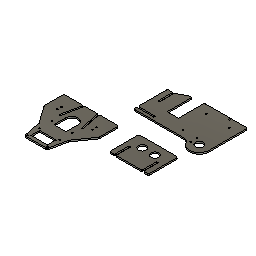
2425-SACBOT-LINE v17 (Autodesk Fusion 360 design; units mm, degrees)
Autodesk Fusion 360 part; units mm, degrees
sketch "Plate Alpha" plane through (0, 0, 0) normal (0, 0, 1) x (1, 0, 0)
  line L0 (0, 0) -> (-55.9249, 0)
  line L1 (-55.9249, 0) -> (-55.9249, -40)
  line L2 (-55.9249, -40) -> (-20.5, -90)
  line L3 (-20.5, -90) -> (0, -90) construction
  line L4 (0, 0) -> (0, -90) construction
  circle A0 centre (-35.9249, -25) radius 1.5
  circle A1 centre (-35.9249, -33) radius 1.5
  line L5 (-35.9249, -25) -> (-35.9249, -33)
  line L6 (0, -59.3106) -> (-20.5, -59.3106) construction
  circle A2 centre (-20.5, -59.3106) radius 1.5
  line L7 (-20.5, -59.3106) -> (-20.5, -84.8106) construction
  circle A3 centre (-20.5, -84.8106) radius 1.5
  line L8 (-23.3833, -41.6168) -> (0, 70.9808) construction
  line L9 (-21.9147, -41.9218) -> (1.4687, 70.6758)
  line L10 (-24.852, -41.3118) -> (-1.4687, 71.2858)
  line L11 (-24.852, -41.3118) -> (-21.9147, -41.9218)
  line L12 (-1.4687, 71.2858) -> (1.4687, 70.6758)
  circle A4 centre (-40.9249, -15) radius 5
  circle A5 centre (20.5, -59.3106) radius 1.5
  line L13 (21.9147, -41.9218) -> (-1.4687, 70.6758)
  line L14 (24.852, -41.3118) -> (1.4687, 71.2858)
  line L15 (24.852, -41.3118) -> (21.9147, -41.9218)
  circle A6 centre (35.9249, -33) radius 1.5
  circle A7 centre (40.9249, -15) radius 5
  line L16 (55.9249, -40) -> (20.5, -90)
  line L17 (20.5, -90) -> (0, -90) construction
  circle A8 centre (20.5, -84.8106) radius 1.5
  line L18 (1.4687, 71.2858) -> (-1.4687, 70.6758)
  circle A9 centre (35.9249, -25) radius 1.5
  circle A10 centre (0, -40) radius 12.5
  line L19 (20.5, -84.8106) -> (0, -84.8106) construction
  line L20 (-20.5, -84.8106) -> (0, -84.8106) construction
  line L21 (-31.6847, -74.2135) -> (-24.852, -41.3118) construction
  line L22 (-21.9147, -41.9218) -> (-29.3153, -77.5578) construction
  line L23 (-23.3833, -41.6168) -> (-30.5, -75.8856) construction
  circle A11 centre (-35.9249, -33) radius 3 construction
  line L24 (-12.5, -63.8106) -> (-12.5, -40)
  line L25 (-12.5, -63.8106) -> (0, -63.8106)
  line L26 (12.5, -63.8106) -> (12.5, -40)
  line L27 (12.5, -63.8106) -> (0, -63.8106)
  line L28 (55.9249, 0) -> (55.9249, -40)
  line L29 (0, 0) -> (55.9249, 0)
  line L30 (23.3833, -41.6168) -> (30.5, -75.8856) construction
  circle A12 centre (-20.5, -84.8106) radius 3 construction
  line L31 (-27.9924, -63.8106) -> (27.9924, -63.8106) construction
  circle A13 centre (-20.5, -59.3106) radius 3 construction
  line L32 (-27.9397, -62.3106) -> (28.362, -62.3106) construction
  line L33 (-37.9924, -65.3106) -> (28.1509, -65.3106) construction
  circle A14 centre (-18.1162, -1.5) radius 1.5
  circle A15 centre (-11.9882, -1.5) radius 1.5
  circle A16 centre (11.9882, -1.5) radius 1.5
  circle A17 centre (18.1162, -1.5) radius 1.5
  line L34 (-20.5, -84.8106) -> (-20.5, -109.8106) construction
  line L35 (-20.5, -109.8106) -> (0, -109.8106) construction
  circle A18 centre (-20.5, -109.8106) radius 1.5
  line L36 (-23.5, -84.8106) -> (-23.5, -112.8106)
  line L37 (-23.5, -112.8106) -> (0, -112.8106)
  line L38 (23.5, -84.8106) -> (23.5, -112.8106)
  line L39 (23.5, -112.8106) -> (0, -112.8106)
  circle A19 centre (20.5, -109.8106) radius 1.5
  circle A20 centre (-20.5, -109.8106) radius 3
  circle A21 centre (20.5, -109.8106) radius 3
  line L40 (-16.75, -88.5606) -> (-16.75, -106.0606)
  line L41 (-16.75, -106.0606) -> (0, -106.0606)
  line L42 (-16.75, -88.5606) -> (0, -88.5606)
  line L43 (16.75, -88.5606) -> (0, -88.5606)
  line L44 (16.75, -88.5606) -> (16.75, -106.0606)
  line L45 (16.75, -106.0606) -> (0, -106.0606)
  line L46 (23.4392, -110.4117) -> (30.5, -75.8856)
  line L47 (-30.5, -75.8856) -> (-23.4392, -110.4117)
  point P0 (-55.9249, 0)
  point P1 (20.5, -84.8106)
  point P2 (-28.3039, -65.3106)
  point P3 (-14.7407, 0)
  point P4 (20.5, -109.8106)
  dimension "d123" = 3
  dimension "d124" = 3
  dimension "d125" = 20
  dimension "d126" = 8
  dimension "d127" = 20.5
  dimension "d128" = 3
  dimension "d129" = 25.5
  dimension "d130" = 3
  dimension "d131" = 1.5
  dimension "d132" = -1.5
  dimension "d133" = 10
  dimension "d135" = 25
  dimension "d136" = 40
  dimension "d137" = 50
  dimension "d143" = 35
  dimension "d144" = 115
  dimension "d146" = 6
  dimension "d147" = 10
  dimension "d148" = 15
  dimension "d149" = 15
  dimension "d150" = 50
  dimension "d165" = 6
  dimension "d167" = 6
  dimension "d168" = -1.5
  dimension "d169" = 1.5
  dimension "d170" = 10
  dimension "d171" = 25
  dimension "d214" = 3
  dimension "d215" = 3
  dimension "d243" = 25
  dimension "d244" = 3
  dimension "d245" = 3
  dimension "d246" = 6
  dimension "d247" = 6
  dimension "d272" = 6.75
  dimension "d274" = 3.75
  dimension "d275" = 6.75
  constraint horizontal L0
  constraint perpendicular L0 L1
  constraint parallel L0 L3
  constraint vertical L4
  constraint coincident L0.start L4.start
  constraint coincident L3.end L4.end
  constraint coincident A0.centre L5.start
  constraint coincident A1.centre L5.end
  constraint vertical L5
  constraint coincident L4 L6.start
  constraint perpendicular L4 L6
  constraint coincident L6.end A2.centre
  constraint perpendicular L6 L7
  constraint coincident L7.end A3.centre
  constraint coincident L4 L8.end
  constraint perpendicular L9 L11
  constraint perpendicular L9 L12
  constraint coincident L8.end L12
  constraint symmetric L1.end L4 L16.start
  constraint symmetric L2.end L4 L16.end
  constraint symmetric L3.end L4 L17.end
  constraint symmetric L4 A1 A6
  constraint symmetric L4 A2 A5
  constraint symmetric L4 L7.end P1
  constraint symmetric L4 A3 A8
  constraint symmetric L4 L9.start L13.start
  constraint symmetric L4 L9.end L13.end
  constraint symmetric L4 L10.start L14.start
  constraint symmetric L4 L10.end L14.end
  constraint symmetric L4 A4 A7
  constraint coincident L2.end L7
  constraint coincident L8.start L11
  constraint symmetric L4 A0 A9
  constraint coincident L4 A10.centre
  constraint coincident L2 L21.start
  constraint coincident L2 L22.end
  constraint collinear L10 L21
  constraint collinear L9 L22
  constraint coincident L2 L23.end
  constraint parallel L22 L23
  constraint coincident P0 L1
  constraint coincident P0 L0
  constraint concentric A1 A11
  constraint coincident A10 L24.end
  constraint tangent A10 L24
  constraint coincident L4 L25.end
  constraint perpendicular L4 L25
  constraint coincident L24.start L25
  constraint vertical L24
  constraint symmetric L4 L24.start L26.start
  constraint symmetric L4 L24.end L26.end
  constraint symmetric L4 L25.end L27.end
  constraint coincident L1 P0
  constraint coincident P0 L0.end
  constraint symmetric L0.start L4 L29.start
  constraint symmetric L4 P0 L28.start
  constraint symmetric L4 L8.start L30.start
  constraint symmetric L4 L23.end L30.end
  constraint concentric A3 A12
  constraint tangent L2 A12
  constraint coincident L23 L31.start
  constraint coincident L30 L31.end
  constraint perpendicular L24 L31
  constraint concentric A2 A13
  constraint horizontal L33
  constraint coincident L2 L33.start
  constraint tangent A13 L32
  constraint coincident L33 P2
  constraint coincident L23 P2
  constraint coincident L8 P3
  constraint coincident L0 P3
  constraint tangent L0 A14
  constraint tangent L10 A14
  constraint tangent L9 A15
  constraint tangent L0 A15
  constraint symmetric L4 A14 A17
  constraint symmetric L4 A15 A16
  constraint perpendicular L20 L34
  constraint perpendicular L34 L35
  constraint coincident L4 L35.end
  constraint coincident L34.end L35.start
  constraint symmetric L4 L34.end P4
  constraint symmetric L4 A18 A19
  constraint symmetric L4 L36.start L38.start
  constraint symmetric L4 L36.end L38.end
  constraint symmetric L4 L37.end L39.end
  constraint concentric A18 A20
  constraint concentric A19 A21
  constraint coincident L25.end L31
  constraint coincident L24.start L25.start
  constraint perpendicular L3 L40
  constraint perpendicular L40 L41
  constraint coincident L4 L42.end
  constraint perpendicular L4 L42
  constraint coincident L4 L41.end
  constraint symmetric L4 L40.start L43.start
  constraint symmetric L4 L40.end L44.end
  constraint symmetric L4 L41.end L45.end
  constraint symmetric L4 L42.end L43.end
  constraint coincident A21 L46.start
  constraint tangent A21 L46
  constraint coincident A20 L47.end
  constraint tangent A20 L47
  measures "d123" diameter of A0
  measures "d124" diameter of A1
  measures "d125" distance of L1 L5
  measures "d126" distance of A0.centre A1.centre
  measures "d127" distance of L6.start L6.end
  measures "d128" diameter of A2
  measures "d129" distance of L6.end L7.end
  measures "d130" diameter of A3
  measures "d133" diameter of A4
  measures "d135" diameter of A10
  measures "d136" distance of P0 L1.end
  measures "d137" vertical distance of L1.end L2.end
  measures "d143" distance of L8.start L23.end
  measures "d144" distance of L8.start L8.end
  measures "d146" diameter of A11
  measures "d147" horizontal distance of L2.end L23.end
  measures "d148" distance of L1 A4.centre
  measures "d149" distance of L0 A4.centre
  measures "d150" distance of L3.end A10.centre
  measures "d165" diameter of A12
  measures "d167" diameter of A13
  measures "d170" horizontal distance of L31.start L33.start
  measures "d171" distance of L0 A0.centre
  measures "d214" diameter of A15
  measures "d215" diameter of A14
  measures "d243" distance of L7.end L34.end
  measures "d244" diameter of A18
  measures "d246" diameter of A20
  measures "d247" diameter of A21
  measures "d272" distance of L36 L40
  measures "d274" distance of L20 L42
  measures "d275" distance of L37 L41
sketch "Plate Gamma" plane through (0, 0, 0) normal (0, 0, 1) x (1, 0, 0)
  line L0 (-279.3639, -68.2725) -> (-160.8639, -68.2725)
  line L1 (-160.8639, -68.2725) -> (-160.8639, -118.2725)
  line L2 (-160.8639, -118.2725) -> (-279.3639, -118.2725)
  line L3 (-279.3639, -118.2725) -> (-279.3639, -68.2725)
  line L4 (-220.1139, -68.2725) -> (-220.1139, -118.2725) construction
  circle A0 centre (-233.1139, -93.2725) radius 8
  line L5 (-233.1139, -85.2725) -> (-220.1139, -85.2725)
  line L6 (-233.1139, -101.2725) -> (-220.1139, -101.2725)
  line L7 (-264.3639, -118.2725) -> (-264.3639, -93.2725)
  line L8 (-262.1639, -120.6703) -> (-262.1639, -95.6703)
  line L9 (-266.5639, -120.6703) -> (-266.5639, -95.6703)
  line L10 (-266.5639, -95.6703) -> (-262.1639, -95.6703)
  line L11 (-279.3639, -93.2725) -> (-160.8639, -93.2725) construction
  circle A1 centre (-207.1139, -93.2725) radius 8
  line L12 (-207.1139, -85.2725) -> (-220.1139, -85.2725)
  line L13 (-207.1139, -101.2725) -> (-220.1139, -101.2725)
  line L14 (-178.0639, -120.6703) -> (-178.0639, -95.6703)
  line L15 (-173.6639, -120.6703) -> (-173.6639, -95.6703)
  line L16 (-173.6639, -95.6703) -> (-178.0639, -95.6703)
  arc A2 (-262.1639, -115.2725) -> (-259.1639, -118.2725) centre (-259.1639, -115.2725) ccw
  arc A3 (-269.5639, -118.2725) -> (-266.5639, -115.2725) centre (-269.5639, -115.2725) ccw
  arc A4 (-181.0639, -118.2725) -> (-178.0639, -115.2725) centre (-181.0639, -115.2725) ccw
  arc A5 (-173.6639, -115.2725) -> (-170.6639, -118.2725) centre (-170.6639, -115.2725) ccw
  line L17 (-39.7924, -33.8106) -> (-39.7924, -93.8106)
  line L18 (-39.7924, -93.8106) -> (39.7924, -93.8106)
  line L19 (39.7924, -93.8106) -> (39.7924, -33.8106)
  line L20 (39.7924, -33.8106) -> (-39.7924, -33.8106)
  circle A6 centre (-12.75, -53.8106) radius 7.925
  line L21 (0, -33.8106) -> (0, -93.8106) construction
  line L22 (-12.75, -45.8856) -> (0, -45.8856)
  line L23 (-12.75, -61.7356) -> (0, -61.7356)
  line L24 (-27.9924, -63.8106) -> (27.9924, -63.8106)
  circle A7 centre (12.75, -53.8106) radius 7.925
  line L25 (12.75, -45.8856) -> (0, -45.8856)
  line L26 (12.75, -61.7356) -> (0, -61.7356)
  line L27 (-4.5784, -44.6359) -> (0, -44.6359)
  line L28 (0, -44.6359) -> (0, -33.8106)
  line L29 (-27.9924, -63.8106) -> (-27.9924, -93.8106) construction
  line L30 (-29.7924, -63.8106) -> (-29.7924, -93.8106)
  line L31 (-26.1924, -63.8106) -> (-26.1924, -93.8106)
  line L32 (-29.7924, -63.8106) -> (-26.1924, -63.8106)
  line L33 (27.9924, -63.8106) -> (27.9924, -93.8106) construction
  line L34 (-26.1924, -63.8106) -> (-12.75, -53.8106)
  circle A8 centre (-24.6924, -92.3106) radius 1.5
  circle A9 centre (-31.2924, -92.3106) radius 1.5
  circle A10 centre (24.6924, -92.3106) radius 1.5
  circle A11 centre (31.2924, -92.3106) radius 1.5
  line L35 (29.7924, -63.8106) -> (29.7924, -93.8106)
  line L36 (26.1924, -63.8106) -> (26.1924, -93.8106)
  line L37 (29.7924, -63.8106) -> (26.1924, -63.8106)
  point P0 (-19.1085, -58.5409)
  dimension "d29" = 2.2
  dimension "d30" = -2.2
  dimension "d31" = 16
  dimension "d32" = 25
  dimension "d33" = 13
  dimension "d34" = 44.25
  dimension "d39" = 15
  dimension "d68" = 3
  dimension "d69" = 6
  dimension "d178" = 15.85
  dimension "d182" = 1.8
  dimension "d183" = -1.8
  dimension "d186" = 10
  dimension "d189" = 60
  dimension "d230" = 3
  dimension "d231" = 3
  dimension "d248" = 20
  dimension "d249" = 30
  dimension "d250" = 25.5
  constraint horizontal L0
  constraint vertical L1
  constraint horizontal L2
  constraint vertical L3
  constraint midpoint L0 L4.start
  constraint midpoint L2 L4.end
  constraint coincident A0 L5.start
  constraint coincident L4 L5.end
  constraint horizontal L5
  constraint tangent A0 L5
  constraint coincident A0 L6.start
  constraint coincident L4 L6.end
  constraint horizontal L6
  constraint tangent A0 L6
  constraint coincident L2 L7.start
  constraint perpendicular L2 L7
  constraint perpendicular L8 L10
  constraint midpoint L3 L11.start
  constraint midpoint L1 L11.end
  constraint coincident A0.centre L11
  constraint coincident L7.end L11
  constraint symmetric L4 A0 A1
  constraint symmetric L4 L5.start L12.start
  constraint symmetric L4 L5.end L12.end
  constraint symmetric L4 L6.start L13.start
  constraint symmetric L4 L6.end L13.end
  constraint symmetric L4 L8.start L14.start
  constraint symmetric L4 L8.end L14.end
  constraint symmetric L4 L9.start L15.start
  constraint symmetric L4 L9.end L15.end
  constraint tangent L2 A2
  constraint tangent L8 A2
  constraint coincident L2 A2.end
  constraint coincident L8 A2.start
  constraint tangent L2 A3
  constraint tangent L9 A3
  constraint coincident L9 A3.end
  constraint coincident L2 A3.start
  constraint symmetric L4 A2.end A4.start
  constraint symmetric L4 A2.start A4.end
  constraint symmetric L4 A2 A4
  constraint symmetric L4 A3.end A5.start
  constraint symmetric L4 A3.start A5.end
  constraint symmetric L4 A3 A5
  constraint vertical L17
  constraint perpendicular L17 L18
  constraint perpendicular L18 L19
  constraint midpoint L20 L21.start
  constraint midpoint L18 L21.end
  constraint perpendicular L18 L21
  constraint coincident A6 L22.start
  constraint coincident L21 L22.end
  constraint tangent A6 L22
  constraint perpendicular L21 L22
  constraint coincident A6 L23.start
  constraint coincident L21 L23.end
  constraint tangent A6 L23
  constraint perpendicular L21 L23
  constraint symmetric A6 L21 A7
  constraint symmetric L21 L22.start L25.start
  constraint symmetric L21 L22.end L25.end
  constraint symmetric L21 L23.start L26.start
  constraint symmetric L21 L23.end L26.end
  constraint horizontal L20
  constraint horizontal L27
  constraint coincident L20 L21.start
  constraint perpendicular L20 L28
  constraint midpoint L21 L24
  constraint coincident L24.start L29.start
  constraint coincident L18 L29.end
  constraint perpendicular L18 L29
  constraint perpendicular L31 L32
  constraint coincident L24.end L33.start
  constraint coincident L18 L33.end
  constraint perpendicular L18 L33
  constraint coincident A6.centre L34.end
  constraint coincident A6 P0
  constraint coincident L34 P0
  constraint coincident L18 L31.end
  constraint coincident L18 L30.end
  constraint tangent L30 A9
  constraint tangent L18 A9
  constraint tangent L31 A8
  constraint tangent L18 A8
  constraint symmetric L21 A8 A10
  constraint symmetric L21 A9 A11
  constraint symmetric L21 L30.start L35.start
  constraint symmetric L21 L30.end L35.end
  constraint symmetric L21 L31.start L36.start
  constraint symmetric L21 L31.end L36.end
  measures "d31" diameter of A0
  measures "d32" distance of L2 A0.centre
  measures "d33" distance of L4 A0.centre
  measures "d34" distance of L4 L7.start
  measures "d39" distance of L7.end L11.start
  measures "d68" radius of A2
  measures "d69" diameter of A3
  measures "d178" diameter of A6
  measures "d186" distance of L17 L30
  measures "d189" distance of L17.start L17.end
  measures "d230" diameter of A8
  measures "d231" diameter of A9
  measures "d248" distance of L20 A6.centre
  measures "d249" distance of L30.start L30.end
  measures "d250" distance of A7.centre A6.centre
sketch "Plate Beta" plane through (0, 0, 0) normal (0, 0, 1) x (1, 0, 0)
  line L0 (48.3507, -123.1753) -> (48.3507, -73.1753)
  line L1 (48.3507, -73.1753) -> (193.8507, -73.1753)
  line L2 (193.8507, -73.1753) -> (193.8507, -146.3349)
  line L3 (68.8507, -146.1753) -> (68.8507, -123.1753)
  line L4 (68.8507, -123.1753) -> (48.3507, -123.1753)
  line L5 (68.8507, -73.1753) -> (68.8507, -98.1753)
  line L6 (66.6507, -73.7918) -> (66.6507, -98.7918)
  line L7 (71.0507, -73.7918) -> (71.0507, -98.7918)
  line L8 (66.6507, -98.7918) -> (71.0507, -98.7918)
  line L9 (68.8507, -123.1753) -> (93.8507, -123.1753)
  line L10 (93.8507, -123.1753) -> (93.8507, -126.1753)
  line L11 (93.8507, -126.1753) -> (68.8507, -126.1753)
  arc A0 (66.6507, -76.1753) -> (63.6507, -73.1753) centre (63.6507, -76.1753) ccw
  arc A1 (74.0507, -73.1753) -> (71.0507, -76.1753) centre (74.0507, -76.1753) ccw
  arc A2 (71.8507, -126.1753) -> (68.8507, -129.1753) centre (71.8507, -129.1753) ccw
  arc A3 (142.4447, -171.4545) -> (193.8507, -146.3349) centre (162.0103, -146.3349) ccw
  line L12 (83.4734, -73.1753) -> (83.4734, -159.2628) construction
  line L13 (83.4734, -116.2191) -> (95.5231, -116.2191) construction
  line L14 (95.5231, -116.2191) -> (180.6062, -116.2191) construction
  circle A4 centre (83.4734, -116.2191) radius 4.5
  line L15 (111.0507, -57.3516) -> (111.0507, -183.7559) construction
  line L16 (93.8507, -123.1753) -> (193.8507, -123.1753) construction
  line L17 (125.0507, -57.3516) -> (125.0507, -183.7559) construction
  line L18 (177.1507, -57.3516) -> (177.1507, -183.7559) construction
  line L19 (95.9516, -120.6753) -> (195.9516, -120.6753) construction
  line L20 (95.9516, -115.5753) -> (195.9516, -115.5753) construction
  line L21 (95.9516, -87.6753) -> (195.9516, -87.6753) construction
  circle A5 centre (125.0507, -120.6753) radius 1.5
  circle A6 centre (177.1507, -115.5753) radius 1.5
  circle A7 centre (177.1507, -87.6753) radius 1.5
  circle A8 centre (159.8734, -146.2859) radius 8
  line L22 (119.02, -178.1753) -> (211.8685, -178.1753)
  arc A9 (142.4447, -171.4545) -> (68.8507, -146.1753) centre (68.8507, -265.9397) ccw
  line L23 (68.8507, -146.1753) -> (95.1653, -146.1753) construction
  line L24 (-23.3833, -41.6168) -> (0, 70.9808)
  line L25 (-23.3833, -41.6168) -> (-30.5, -75.8856)
  circle A10 centre (171.8682, 109.4824) radius 1.5
  circle A11 centre (123.6682, 110.7824) radius 1.5
  circle A12 centre (128.7682, 58.6824) radius 1.5
  circle A13 centre (156.6682, 58.6824) radius 1.5
  line L26 (156.6682, 58.6824) -> (128.7682, 58.6824) construction
  line L27 (174.4682, 124.7824) -> (121.1682, 124.7824) construction
  line L28 (121.1682, 124.7824) -> (121.1682, 56.1824) construction
  line L29 (121.1682, 56.1824) -> (174.4682, 56.1824) construction
  line L30 (174.4682, 56.1824) -> (174.4682, 124.7824) construction
  line L31 (-39.7924, -33.8106) -> (-39.7924, -93.8106)
  line L32 (-27.9924, -63.8106) -> (-27.9924, -93.8106)
  line L33 (41.1416, 114.4163) -> (41.1416, 54.4163)
  line L34 (41.1416, 54.4163) -> (76.1416, 54.4163)
  line L35 (76.1416, 54.4163) -> (76.1416, 51.4163)
  line L36 (76.1416, 51.4163) -> (41.1416, 51.4163)
  line L37 (41.1416, 51.4163) -> (41.1416, 29.4163)
  line L38 (41.1416, 114.4163) -> (51.8242, 114.4163)
  line L39 (51.8242, 114.4163) -> (51.8242, 84.4163)
  line L40 (51.8242, 84.4163) -> (55.1242, 84.4163)
  line L41 (55.1242, 84.4163) -> (55.1242, 114.4163)
  line L42 (191.1416, 127.4163) -> (191.1416, 29.4163)
  line L43 (55.1242, 114.4163) -> (80.2572, 127.4163)
  line L44 (80.2572, 127.4163) -> (191.1416, 127.4163)
  line L45 (191.1416, 29.4163) -> (41.1416, 29.4163)
  line L46 (118.6464, 29.4163) -> (118.6464, 127.4163) construction
  circle A14 centre (171.1416, 49.4163) radius 20
  line L47 (41.1416, 45.4163) -> (143.7995, 45.4163)
  arc A15 (153.7053, 39.6197) -> (143.7995, 45.4163) centre (143.7995, 34.0541) ccw
  circle A16 centre (56.6242, 113.5034) radius 1.5
  circle A17 centre (50.3242, 112.9163) radius 1.5
  circle A18 centre (171.1416, 49.4163) radius 8
  line L48 (80.2572, 127.4163) -> (80.2572, 74.4163)
  line L49 (80.2572, 74.4163) -> (103.2572, 74.4163)
  line L50 (103.2572, 74.4163) -> (103.2572, 127.4163)
  line L51 (157.2609, 45.7074) -> (157.2609, 123.8574) construction
  circle A19 centre (157.2609, 45.7074) radius 1.5
  circle A20 centre (157.2609, 45.7074) radius 5.9 construction
  circle A21 centre (157.2609, 123.8574) radius 1.5
  circle A22 centre (157.2609, 123.8574) radius 5.9 construction
  line L52 (130.7609, 44.7824) -> (183.7609, 44.7824) construction
  line L53 (183.7609, 44.7824) -> (183.7609, 124.7824) construction
  line L54 (183.7609, 124.7824) -> (130.7609, 124.7824) construction
  line L55 (130.7609, 124.7824) -> (130.7609, 44.7824) construction
  line L56 (130.7609, 44.7824) -> (183.7609, 124.7824) construction
  point P0 (53.4742, 84.4163)
  point P1 (-14.7407, 0)
  point P2 (41.1416, 45.4163)
  dimension "d17" = 2.2
  dimension "d18" = -2.2
  dimension "d19" = 25
  dimension "d20" = 50
  dimension "d21" = 3
  dimension "d22" = 25
  dimension "d25" = 20.5
  dimension "d26" = 20.5
  dimension "d27" = 100
  dimension "d28" = 20
  dimension "d64" = 3
  dimension "d65" = 6
  dimension "d66" = 3
  dimension "d80" = 9
  dimension "d81" = 40
  dimension "d82" = -14
  dimension "d83" = -66.1
  dimension "d84" = -2.5
  dimension "d85" = -7.6
  dimension "d86" = -35.5
  dimension "d87" = 3
  dimension "d88" = 3
  dimension "d89" = 3
  dimension "d90" = 16
  dimension "d115" = 55
  dimension "d151" = 3
  dimension "d152" = 3
  dimension "d153" = 3
  dimension "d154" = 3
  dimension "d157" = 27.9
  dimension "d160" = 68.6
  dimension "d161" = 53.3
  dimension "d162" = 2.5
  dimension "d163" = 14
  dimension "d190" = 115
  dimension "d191" = 35
  dimension "d192" = 60
  dimension "d193" = 30
  dimension "d195" = 12.3326
  dimension "d196" = 12.3326
  dimension "d197" = 3.3
  dimension "d198" = 115
  dimension "d199" = 60
  dimension "d200" = 30
  dimension "d202" = 3
  dimension "d203" = 25
  dimension "d204" = 72.4953
  dimension "d205" = 72.4953
  dimension "d206" = 6
  dimension "d207" = 3
  dimension "d208" = 3
  dimension "d211" = 35
  dimension "d212" = 40
  dimension "d213" = 16
  dimension "d251" = 23
  dimension "d252" = 53
  dimension "d253" = 20
  dimension "d256" = 5.1
  dimension "d257" = 15.2
  dimension "d258" = 1.3
  dimension "d259" = 50.8
  dimension "d260" = 78.15
  dimension "d261" = 80
  dimension "d262" = 3
  dimension "d263" = 11.8
  dimension "d264" = 3
  dimension "d265" = 11.8
  dimension "d266" = 53
  dimension "d267" = 180
  constraint vertical L0
  constraint perpendicular L0 L1
  constraint perpendicular L1 L2
  constraint parallel L2 L3
  constraint horizontal L4
  constraint coincident L1 L5.start
  constraint perpendicular L1 L5
  constraint perpendicular L7 L8
  constraint perpendicular L3 L9
  constraint perpendicular L9 L10
  constraint coincident L3 L11.end
  constraint horizontal L11
  constraint tangent L1 A0
  constraint tangent L6 A0
  constraint coincident L1 A0.end
  constraint coincident L6 A0.start
  constraint tangent L7 A1
  constraint tangent L1 A1
  constraint coincident L7 A1.end
  constraint coincident L1 A1.start
  constraint tangent L3 A2
  constraint tangent L11 A2
  constraint coincident L3 A2.end
  constraint coincident L11 A2.start
  constraint tangent L2 A3
  constraint coincident L1 L12.start
  constraint perpendicular L1 L12
  constraint midpoint L12 L13.start
  constraint perpendicular L12 L13
  constraint perpendicular L12 L14
  constraint coincident L13.start A4.centre
  constraint vertical L15
  constraint coincident L2 L16.end
  constraint horizontal L16
  constraint coincident L17 A5.centre
  constraint coincident L19 A5.centre
  constraint coincident L20 A6.centre
  constraint coincident L18 A6.centre
  constraint coincident L21 A7.centre
  constraint coincident L18 A7.centre
  constraint horizontal L22
  constraint tangent A3 L22
  constraint tangent A3 A9
  constraint perpendicular L3 L23
  constraint tangent A9 L23
  constraint coincident A13.centre L26.start
  constraint coincident A12.centre L26.end
  constraint perpendicular L27 L28
  constraint perpendicular L28 L29
  constraint coincident L27.start L30.end
  constraint vertical L18
  constraint vertical L33
  constraint perpendicular L33 L34
  constraint perpendicular L34 L35
  constraint perpendicular L35 L36
  constraint perpendicular L36 L37
  constraint perpendicular L33 L38
  constraint perpendicular L38 L39
  constraint perpendicular L33 L40
  constraint perpendicular L38 L41
  constraint perpendicular L38 L42
  constraint midpoint L40 P0
  constraint collinear L33 L37
  constraint coincident L42.start L44.end
  constraint horizontal L44
  constraint coincident L38 L41.end
  constraint perpendicular L42 L45
  constraint coincident L37.end L45.end
  constraint coincident L45 L46.start
  constraint coincident L44 L46.end
  constraint perpendicular L44 L46
  constraint coincident L37 P2
  constraint tangent L42 A14
  constraint tangent L45 A14
  constraint coincident P2 L47.start
  constraint perpendicular L37 L47
  constraint coincident A14 A15.start
  constraint tangent L47 A15
  constraint tangent A14 A15
  constraint tangent L41 A16
  constraint tangent L43 A16
  constraint tangent L39 A17
  constraint tangent L38 A17
  constraint coincident A14.centre A18.centre
  constraint coincident L44 L43.end
  constraint perpendicular L44 L48
  constraint perpendicular L41 L49
  constraint coincident L44 L50.end
  constraint perpendicular L44 L50
  constraint coincident L43.end L48
  constraint perpendicular L27 L30
  constraint vertical L30
  constraint parallel L26 L29
  constraint coincident L51.start A19.centre
  constraint concentric A19 A20
  constraint coincident L51.end A21.centre
  constraint concentric A21 A22
  constraint perpendicular L53 L54
  constraint midpoint L51 L56
  constraint perpendicular L52 L55
  constraint perpendicular L54 L55
  constraint parallel L51 L55
  measures "d19" distance of L5.start L5.end
  measures "d20" distance of L0.start L0.end
  measures "d21" distance of L9.end L10.end
  measures "d22" distance of L10.end L11.end
  measures "d25" distance of L0.start L3.end
  measures "d26" distance of L0 L5
  measures "d27" distance of L2 L9.end
  measures "d28" distance of L3.start L11.end
  measures "d64" radius of A0
  measures "d65" diameter of A1
  measures "d66" radius of A2
  measures "d80" diameter of A4
  measures "d81" distance of L7 L15
  measures "d87" diameter of A5
  measures "d88" diameter of A6
  measures "d89" diameter of A7
  measures "d90" diameter of A8
  measures "d115" distance of L9.end L22
  measures "d151" diameter of A10
  measures "d152" diameter of A11
  measures "d153" diameter of A12
  measures "d154" diameter of A13
  measures "d157" distance of A13.centre A12.centre
  measures "d160" distance of L27.end L28.end
  measures "d161" distance of L27.start L27.end
  measures "d162" distance of A11.centre L28
  measures "d163" distance of A11.centre L27
  measures "d190" distance of L24.start L24.end
  measures "d191" distance of L24.start L25.end
  measures "d192" distance of L31.start L31.end
  measures "d193" distance of L32.start L32.end
  measures "d195" distance of L25.end L32.start
  measures "d196" distance of L33 P0
  measures "d197" distance of L39 L41
  measures "d198" distance of L35 L42
  measures "d199" distance of L33.start L33.end
  measures "d200" distance of L38.end L39.end
  measures "d202" distance of L34 L36
  measures "d203" distance of L34 L42.end
  measures "d204" distance of L24.end P1
  measures "d205" distance of L42 L46
  measures "d206" distance of L36.end P2
  measures "d207" diameter of A16
  measures "d208" diameter of A17
  measures "d211" distance of L35.end L36.end
  measures "d212" diameter of A14
  measures "d213" diameter of A18
  measures "d251" distance of L48 L50
  measures "d252" distance of L44 L49
  measures "d253" distance of L34 L49
  measures "d256" horizontal distance of A11.centre A12.centre
  measures "d257" horizontal distance of A10.centre A13.centre
  measures "d258" vertical distance of A10.centre A11.centre
  measures "d259" vertical distance of A10.centre A13.centre
  measures "d260" distance of L51.start L51.end
  measures "d261" distance of L52.start L54.end
  measures "d262" diameter of A19
  measures "d263" diameter of A20
  measures "d264" diameter of A21
  measures "d265" diameter of A22
  measures "d266" distance of L53.end L54.end
  measures "d267" angle of L42 L55
extrude "Extrude6" add sketch "Plate Alpha" along normal blind 3 contours L0 L1 L2 L9 L10 L11 L13 L14 L15 L16 L28 L29 A14 A15 A16 A17 L36 L37 L38 L39 A20 A21 | A15 | A16 | A14 | A17 | L2 L36 L47 | L16 L38 L46 | L36 A20 L47 | L38 A21 L46 | A20 | A21 | A4 | A7 makes body 1
extrude "Extrude7" add sketch "Plate Beta" along normal blind 3 separate body contours L33 L34 L35 L36 L37 L38 L39 L40 L41 L42 L43 L44 A14 L47 A15 A16 A17 L48 L49 L50 | A17 | A16 | A14 makes body 2
extrude "Extrude8" add sketch "Plate Gamma" along normal blind 3 separate body contours L17 L18 L19 L20 L24 L30 L32 A9 A11 L35 L37 | A9 | A11 | L18 L24 L31 A8 A10 L36 | A8 | A10 | A6 L22 L23 A7 L25 L26 makes body 3
fillet "Fillet1" radius 3 17 edges at (12.5, -63.8106, 1.5) (-12.5, -63.8106, 1.5) (-55.9249, 0, 1.5) (55.9249, 0, 1.5) (55.9249, -40, 1.5) (-55.9249, -40, 1.5) (80.2572, 127.4163, 1.5) (103.2572, 127.4163, 1.5) (41.1416, 54.4163, 1.5) (41.1416, 51.4163, 1.5) (41.1416, 45.4163, 1.5) (41.1416, 114.4163, 1.5) (191.1416, 127.4163, 1.5) (39.7924, -33.8106, 1.5) (-39.7924, -33.8106, 1.5) (39.7924, -93.8106, 1.5) (-39.7924, -93.8106, 1.5) on bodies 1 2 3
move_body "Move2" bodies 3 to x (1, 0, 0) y (0, 1, 0) z (0, 0, 1) at (131.553, 39.2045, 0)
fillet "Fillet2" [no effect]
copy_body "Body->Comp5" [suppressed] in component "Component"
copy_body "Body->Comp6" [suppressed] in component "Component'"
copy_body "Body->Comp7" [suppressed] in component "Component''"
extrude "Extrude2" [suppressed]
extrude "Extrude3" [suppressed]
extrude "Extrude4" [suppressed]
copy_body "Body->Comp2" [suppressed] in component "MainBody"
copy_body "Body->Comp3" [suppressed] in component "VerticalFin/Tail"
copy_body "Body->Comp4" [suppressed] in component "VerticalFront"
equation "d1 = ( 3 / 2 ) * 1 mm"
equation "d9 = 40 mm"
equation "d16 = 60 mm"
equation "d20 = 2 * d19"
equation "d21 = 2 * d1"
equation "d27 = d16 + d9"
equation "d32 = d19"
equation "d33 = ( 42 mm - d31 ) / 2"
equation "d83 = -14 mm - 1.3 mm - 50.8 mm"
equation "d85 = -2.5 mm - 5.1 mm"
equation "d86 = -2.5 mm - 5.1 mm - 27.9 mm"
equation "d132 = -d131"
equation "d145 = 6 mm"
equation "d146 = d145"
equation "d152 = d151"
equation "d153 = d151"
equation "d154 = d151"
equation "d178 = 16 mm - 0.15 mm"
equation "d182 = ( 3.6 / 2 ) * 1 mm"
equation "d183 = -d182"
equation "d196 = d195"
equation "d198 = d190"
equation "d199 = d192"
equation "d200 = d193"
equation "d205 = d204"
equation "d211 = d191"
equation "d250 = 41.5 mm - 16 mm"
equation "d272 = d245 - 2.25 mm + 6 mm"
equation "d274 = 6 mm - 2.25 mm"
equation "d275 = d272"
